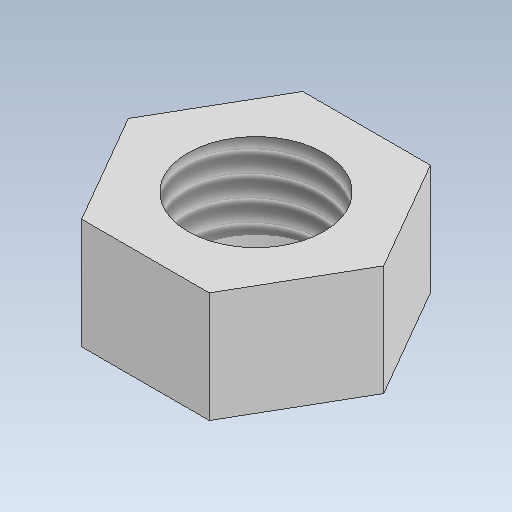
# Autodesk Inventor part: M8_nut_6.5mm
Saved by Autodesk Inventor 2020.3 (Build 243373000, 373)
## iProperties
Created: 2021-03-23
Part Number: M8_nut_6.5mm
Material: Ogólny
Document SubType Name: Modeling
Designer: patry
Density: 1 g/cm^3
Appearance: Domyślna
Author: patry
Autodesk Inventor part; units mm, degrees
ref_plane "YZ Plane" through (0, 0, 0) normal (1, 0, 0) x (0, 1, 0)
ref_plane "XZ Plane" through (0, 0, 0) normal (0, 1, 0) x (-1, 0, 0)
ref_plane "XY Plane" through (0, 0, 0) normal (0, 0, 1) x (1, 0, 0)
sketch "Szkic1" plane through (0, 0, 0) normal (0, 1, 0) x (-1, 0, 0)
  line L0 (-3.7528, -6.5) -> (-7.5056, 0)
  line L1 (-7.5056, 0) -> (-3.7528, 6.5)
  line L2 (-3.7528, 6.5) -> (3.7528, 6.5)
  line L3 (3.7528, 6.5) -> (7.5056, 0)
  line L4 (7.5056, 0) -> (3.7528, -6.5)
  line L5 (3.7528, -6.5) -> (-3.7528, -6.5)
  circle A0 centre (0, 0) radius 4
  dimension "d0" = 13
  dimension "d1" = 8
  constraints: 12 end point, 2 coincident, 1 centre point, 13 other
  measures "d0" distance between parallel lines of L2 L5
  measures "d1" diameter of A0
extrude "Wyciągnięcie proste1" add sketch "Szkic1" along normal blind 6.5
thread "Gwint1" size "M8x1.25" class "6H" standard "ANSI Metric M Profile" length 5
